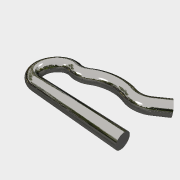
# Autodesk Inventor part: PWTR-0114
Saved by Autodesk Inventor 2021.1 (Build 251245000, 245)
## iProperties
Created: 2020-09-01
Part Number: PWTR-0114
Material: Steel, High Strength, Low Alloy
Document SubType Name: Modeling
Designer: alid
Density: 7.85 g/cm^3
Appearance: Steel - Polished
Description: Arm Pivot Clevis Pin
Author: alid
Revision Number: A
Autodesk Inventor part; units mm, degrees
ref_plane "YZ Plane" through (0, 0, 0) normal (1, 0, 0) x (0, 1, 0)
ref_plane "XZ Plane" through (0, 0, 0) normal (0, 1, 0) x (-1, 0, 0)
sketch "Sketch1" plane through (0, 0, 0) normal (0, 0, 1) x (1, 0, 0)
  line L0 (0, -9.5) -> (0, 9.5)
  arc A0 (7.7897, 8.2201) -> (0, 9.5) centre (4, 9.5) ccw
  circle A1 centre (0, 0) radius 9.5 construction
  arc A2 (7.7897, 8.2201) -> (8.1485, 4.8839) centre (11.5794, 6.9402) ccw
  arc A3 (8.6168, -4) -> (8.1485, 4.8839) centre (0, 0) ccw
  arc A4 (8.6168, -4) -> (8.9684, -7.9785) centre (12.245, -5.6842) ccw
  line L1 (8.9684, -7.9785) -> (10.6891, -10.436)
  circle A5 centre (0, 0) radius 8 construction
  dimension "d0" = 19
  dimension "d1" = 19
  dimension "d2" = 4
  dimension "d3" = 4
  dimension "d4" = 4
  dimension "d7" = 3
  dimension "d8" = 4
  dimension "d12" = 16
  dimension "d13" = 35
  constraints: 8 point on circle, 6 centre point, 5 tangent, 4 end point, 3 coincident, 2 concentric, 1 midpoint, 1 vertical
  measures "d0" distance of L0.start L0.end
  measures "d1" diameter of A1
  measures "d2" radius of A2
  measures "d3" radius of A0
  measures "d4" radius of A4
  measures "d7" distance of L1.start L1.end
  measures "d8" vertical distance of A3.start point (0, 0)
  measures "d12" diameter of A5
  measures "d13" angle of L0 L1
ref_plane "Work Plane1" through (0, -9.5, 0) normal (0, 1, 0) x (-1, 0, 0)
sketch "Sketch2" plane through (0, -9.5, 0) normal (0, 1, 0) x (-1, 0, 0)
  circle A0 centre (0, 0) radius 1.5
  point P0 (0, 0)
  dimension "d9" = 3
  constraints: 1 centre point, 1 coincident
  measures "d9" diameter of A0
sweep "Sweep1" add profiles "Sketch2" path "Sketch1"
equation "\"d0\" = d1"
equation "\"d4\" = d2"
equation "\"d8\" = d3"
body "Solid1"
